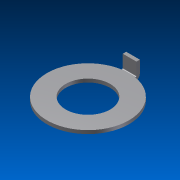
# Autodesk Inventor part: SPDT Toggle Switch Anti-Rotation Washer
Saved by Autodesk Inventor 2011 SP1 (Build 150282100, 282)
## iProperties
Created: 2011-11-07
Part Number: SPDT Toggle Switch Anti-Rotation Washer
Document SubType Name: Modeling
Designer: sdarley
Density: 1 g/cm^3
Author: sdarley
Autodesk Inventor part; units mm, degrees
ref_plane "YZ Plane" through (0, 0, 0) normal (1, 0, 0) x (0, 1, 0)
ref_plane "XZ Plane" through (0, 0, 0) normal (0, 1, 0) x (-1, 0, 0)
ref_plane "XY Plane" through (0, 0, 0) normal (0, 0, 1) x (1, 0, 0)
sketch "Sketch1" plane through (0, 0, 0) normal (0, 0, 1) x (1, 0, 0)
  circle A0 centre (0, 0) radius 6
  circle A1 centre (0, 0) radius 3.25
  dimension "d0" = 12
  dimension "d1" = 6.5
  constraints: 2 centre point, 2 coincident
  measures "d0" diameter of A0
  measures "d1" diameter of A1
extrude "Extrusion1" add sketch "Sketch1" along normal blind 0.5
sketch "Sketch2" plane through (0, 0, 0) normal (1, 0, 0) x (0, 1, 0)
  line L0 (-6, 0.5) -> (6, 0.5) projected
  line L1 (-6, 0) -> (6, 0) projected
  line L2 (6, 0) -> (6, 0.5) projected
  line L3 (6.1, 0.6) -> (6.1, 2.4)
  line L4 (6.1, 2.4) -> (6.6, 2.4)
  line L5 (6.6, 2.4) -> (6.6, 0.6)
  arc A0 (6, 0.5) -> (6.1, 0.6) centre (6, 0.6) ccw
  arc A1 (6, 0) -> (6.6, 0.6) centre (6, 0.6) ccw
  line L6 (6, 0.5) -> (6, 0)
  point P0 (0, 0)
  dimension "d6" = 0.2
  dimension "d7" = 0.5
  dimension "d8" = 2.4
  constraints: 9 end point, 4 point on circle, 2 centre point, 2 equal length, 2 tangent, 1 coincident
  measures "d6" diameter of A0
  measures "d7" distance between parallel lines of L5 L3
  measures "d8" distance between parallel lines of L1 L4
extrude "Extrusion2" add sketch "Sketch2" along normal mid plane 2
sketch "Sketch3" plane through (0, 0, 0) normal (0, 0, -1) x (-1, 0, 0)
  circle A0 centre (0, 0) radius 6 projected
  line L0 (-1, 6.6) -> (-1, 6) projected
  line L1 (-1, 6) -> (0, 6) projected
  line L2 (0, 6) -> (1, 6) projected
  line L3 (1, 6) -> (1, 6.6) projected
  line L4 (1, 6.6) -> (-1, 6.6) projected
  line L5 (-1, 6) -> (-1, 5.9161)
  line L6 (1, 6) -> (1, 5.9161)
  constraints: 4 end point, 2 point on circle, 1 parallel, 1 perpendicular
extrude "Extrusion3" add sketch "Sketch3" against normal up to surface (0.5 mm away) contours A0 L2 L6 | L5 L1 A0
body "Solid1"
